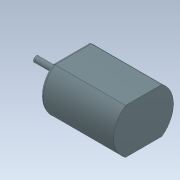
# Autodesk Inventor part: Motor
Saved by Autodesk Inventor 2021 (Build 250183000, 183)
## iProperties
Created: 2021-08-29
Part Number: Motor
Material: Iron, Cast
Document SubType Name: Modeling
Designer: digge
Density: 7.15 g/cm^3
Appearance: Lead
Author: digge
Autodesk Inventor part; units mm, degrees
ref_plane "YZ Plane" through (0, 0, 0) normal (1, 0, 0) x (0, 1, 0)
ref_plane "XZ Plane" through (0, 0, 0) normal (0, 1, 0) x (-1, 0, 0)
ref_plane "XY Plane" through (0, 0, 0) normal (0, 0, 1) x (1, 0, 0)
sketch "Sketch3" plane through (0, 0, 0) normal (1, 0, 0) x (0, 1, 0)
  line L0 (23.8462, 26.7077) -> (8.4462, 26.7077) construction
  line L1 (8.4462, 26.7077) -> (8.4462, 14.3077)
  line L2 (8.4462, 14.3077) -> (23.8462, 14.3077) construction
  line L3 (23.8462, 14.3077) -> (23.8462, 26.7077)
  line L4 (16.1462, 26.7077) -> (16.1462, 30.7077) construction
  line L5 (16.1462, 14.3077) -> (16.1462, 10.3077) construction
  arc A0 (8.4462, 14.3077) -> (23.8462, 14.3077) centre (16.1462, 19.7189) ccw
  arc A1 (23.8462, 26.7077) -> (8.4462, 26.7077) centre (16.1462, 21.2964) ccw
  point P0 (0, 0)
  dimension "d9" = 12.4
  dimension "d10" = 15.4
  dimension "d11" = 4
  dimension "d12" = 4
  dimension "d13" = 20.4
  constraints: 12 end point, 6 point on circle, 2 centre point, 2 midpoint, 2 perpendicular, 2 vertical
  measures "d9" distance of L2.end L0.start
  measures "d10" distance of L1.end L2.end
  measures "d11" distance of L4.start L4.end
  measures "d12" distance of L5.start L5.end
  measures "d13" distance of L5.end L4.end
extrude "Extrusion1" add sketch "Sketch3" along normal blind 25.1
sketch "Sketch4" plane through (0, 0, 0) normal (-1, 0, 0) x (0, 0, 1)
  line L0 (26.7077, 8.4462) -> (14.3077, 8.4462) projected
  line L1 (14.3077, 23.8462) -> (26.7077, 23.8462) projected
  arc A0 (14.3077, 23.8462) -> (14.3077, 8.4462) centre (19.7189, 16.1462) ccw projected
  arc A1 (26.7077, 8.4462) -> (26.7077, 23.8462) centre (21.2964, 16.1462) ccw projected
  circle A2 centre (20.5077, 16.1462) radius 3.075
  point P0 (0, 0)
  dimension "d16" = 6.15
  constraints: 1 centre point
  measures "d16" diameter of A2
extrude "Extrusion2" add sketch "Sketch4" along normal blind 1.6 contours A2
sketch "Sketch5" plane through (-1.6, 16.1462, 20.5077) normal (-1, 0, 0) x (0, 0, 1)
  circle A0 centre (0, 0) radius 1
  point P0 (-20.5077, -16.1462)
  dimension "d19" = 2
  constraints: 1 centre point
  measures "d19" diameter of A0
extrude "Extrusion3" add sketch "Sketch5" along normal blind 9.95
fillet "Fillet3" radius 1 5 edges at (-1.6, 16.1462, 17.4327) (0, 23.8462, 20.5077) (0, 16.1462, 30.7077) (0, 8.4462, 20.5077) (0, 16.1462, 10.3077)
body "Solid2"
